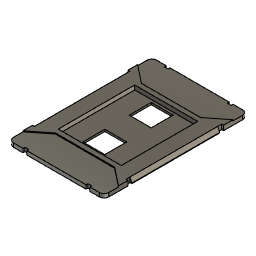
Clipsal Iconic Grid - 2 Gang (Autodesk Fusion 360 design; units mm, degrees)
Autodesk Fusion 360 part; units mm, degrees
note: some values were not read from the file. Set by a fixed rule: which sketch regions a step uses.
sketch "Body Quarter" plane through (0, 0, 0) normal (0, 0, 1) x (1, 0, 0)
  arc A0 (-45, 75) -> (-50, 70) centre (-45, 70) ccw
  line L0 (-50, 50) -> (-48, 50)
  line L1 (-48, 50) -> (-48, 46)
  line L2 (-48, 46) -> (-50, 46)
  line L3 (-50, 70) -> (-50, 50)
  line L4 (0, 0) -> (0, 75)
  line L5 (0, 0) -> (-50, 0)
  line L6 (-50, 46) -> (-50, 0)
  line L7 (-31, 75) -> (-31, 73)
  line L8 (-31, 73) -> (-35, 73)
  line L9 (-35, 73) -> (-35, 75)
  line L10 (0, 75) -> (-31, 75)
  line L11 (-35, 75) -> (-45, 75)
  dimension "d12" = 2
  dimension "d13" = 4
  dimension "d14" = 25
  dimension "d16" = 50
  dimension "d25" = 4
  dimension "d26" = 2
  dimension "d27" = 15
  dimension "d28" = 75
  dimension "d50" = 5
  constraint coincident L5.end L3
  constraint tangent A0 L3
  constraint coincident L2.end L3
  constraint coincident L4.start L5.start
  constraint horizontal L10
  constraint vertical L4
  constraint horizontal L0
  constraint vertical L1
  constraint horizontal L2
  constraint vertical L7
  constraint horizontal L8
  constraint vertical L9
  constraint coincident L9.end L10
  constraint collinear L10 L11
  constraint tangent A0 L11
  constraint horizontal L5
  measures "d12" distance of L0.start L0.end
  measures "d13" distance of L0.end L1.end
  measures "d14" distance of L0.end L10
  measures "d16" distance of L4 L6
  measures "d25" distance of L7.end L8.end
  measures "d26" distance of L9.end L8.end
  measures "d27" distance of L3 L9
  measures "d28" distance of L4.start L10
  measures "d50" radius of A0
extrude "Extrude1" add sketch "Body Quarter" along normal blind 5
chamfer "Chamfer4" distance 4.5 distance2 2 1 edges at (-50, 23, 5) measured on face at (-50, 30.6667, 3.3333)
sketch "Sketch4" plane through (0, 0, 5) normal (0, 0, 1) x (-1, 0, 0)
  line L0 (48, -46) -> (48, 0)
  line L1 (48, 0) -> (0, 0)
  line L2 (0, 0) -> (0, -75)
  line L3 (0, -75) -> (31, -75)
  line L4 (31, -75) -> (31, -73)
  line L5 (31, -73) -> (35, -73)
  line L6 (35, -73) -> (35, -75)
  line L7 (35, -75) -> (45, -75)
  arc A0 (45, -75) -> (50, -70) centre (45, -70) ccw
  line L8 (50, -70) -> (50, -50)
  line L9 (50, -50) -> (48, -50)
  line L10 (48, -50) -> (48, -46)
  line L11 (0, 0) -> (33, 0)
  line L12 (33, 0) -> (33, -40)
  line L13 (33, -40) -> (0, -40)
  line L14 (0, -40) -> (0, 0)
  dimension "d57" = 40
  dimension "d58" = 33
  constraint horizontal L11
  constraint vertical L12
  constraint horizontal L13
  constraint vertical L14
  constraint coincident L1.end L2.start
  measures "d57" distance of L1.end L13.end
  measures "d58" distance of L1.end L11.end
extrude "Extrude4" cut sketch "Sketch4" against normal blind 3 contours L1 L2 L11 L12 L13 L14
chamfer "Chamfer5" distance 3 distance2 1.5 2 edges at (-33, 20, 2) (-16.5, 40, 2) measured on face at (-33, 13.3333, 4) measured on face at (-22, 40, 4)
sketch "Sketch5" plane through (0, 0, 5) normal (0, 0, 1) x (-1, 0, 0)
  line L0 (33, -40) -> (0, -40)
  line L1 (0, -40) -> (0, -75)
  line L2 (0, -75) -> (31, -75)
  line L3 (31, -75) -> (31, -73)
  line L4 (31, -73) -> (35, -73)
  line L5 (35, -73) -> (35, -75)
  line L6 (35, -75) -> (45, -75)
  arc A0 (45, -75) -> (50, -70) centre (45, -70) ccw
  line L7 (50, -70) -> (50, -50)
  line L8 (50, -50) -> (48, -50)
  line L9 (48, -50) -> (48, -46)
  line L10 (48, -46) -> (48, 0)
  line L11 (48, 0) -> (33, 0)
  line L12 (33, 0) -> (33, -40)
  line L13 (0, -45) -> (31, -45)
  line L14 (31, -45) -> (50, -60)
  constraint coincident L1 L13.start
  constraint perpendicular L1 L13
  constraint midpoint L7 L14.end
extrude "Extrude5" cut sketch "Sketch5" against normal blind 1 contours L1 L2 L3 L4 L5 L6 A0 L7 L13 L14
mirror "Mirror1" about plane through (0, 0, 0) normal (1, 0, 0) of bodies 1 merged
mirror "Mirror2" about plane through (0, 0, 0) normal (0, -1, 0) of bodies 1 merged
sketch "Mech Hole" plane through (0, 0, 5) normal (0, 0, 1) x (-1, 0, 0)
  line L0 (50, -60) -> (50, -50)
  line L1 (50, -50) -> (48, -50)
  line L2 (48, -50) -> (48, -46)
  line L3 (48, 46) -> (48, 50)
  line L4 (48, 50) -> (50, 50)
  line L5 (50, 50) -> (50, 60)
  line L6 (-50, 60) -> (-50, 50)
  line L7 (-50, 50) -> (-48, 50)
  line L8 (-48, 50) -> (-48, 46)
  line L9 (-48, -46) -> (-48, -50)
  line L10 (-48, -50) -> (-50, -50)
  line L11 (-50, -50) -> (-50, -60)
  line L12 (-11.5, -35.7841) -> (11.5, -35.7841)
  line L13 (11.5, -35.7841) -> (11.5, -12.7841)
  line L14 (11.5, -12.7841) -> (-11.5, -12.7841)
  line L15 (-11.5, -12.7841) -> (-11.5, -35.7841)
  line L16 (-11.5, -35.7841) -> (11.5, -12.7841) construction
  line L17 (11.5, -35.7841) -> (-11.5, -12.7841) construction
  line L18 (48, -46) -> (48, 46)
  line L19 (-48, 46) -> (-48, -46)
  line L20 (-50, -60) -> (-31, -45)
  line L21 (-31, -45) -> (31, -45)
  line L22 (31, -45) -> (50, -60)
  line L23 (50, 60) -> (31, 45)
  line L24 (31, 45) -> (-31, 45)
  line L25 (-31, 45) -> (-50, 60)
  line L26 (-33, -40) -> (-33, 40)
  line L27 (-33, 40) -> (33, 40)
  line L28 (33, 40) -> (33, -40)
  line L29 (33, -40) -> (-33, -40)
  point P0 (0, -24.2841)
  dimension "d39" = 23
  constraint horizontal L12
  constraint perpendicular L12 L13
  constraint parallel L12 L14
  constraint parallel L13 L15
  constraint coincident L16 P0
  constraint coincident L17 P0
  constraint vertical origin P0
  constraint equal L12 L15
  measures "d39" distance of L12.start L12.end
extrude "Extrude2" cut sketch "Mech Hole" against normal through all contours L12 L13 L14 L15
mirror "Mirror3" about plane through (0, 0, 0) normal (0, 1, 0) of "Extrude2"
equation "d16 = ( 100 / 2 ) * 1 mm"
equation "d28 = ( 150 / 2 ) * 1 mm"
